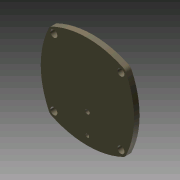
# Autodesk Inventor part: Between Seal 1764
Saved by Autodesk Inventor 2011 (Build 150239000, 239)
## iProperties
Created: 2010-01-18
Part Number: Between Seal 1764
Document SubType Name: Modeling
Designer: wbridges
Density: 1 g/cm^3
Author: wbridges
Autodesk Inventor part; units mm, degrees
ref_plane "YZ Plane" through (0, 0, 0) normal (1, 0, 0) x (0, 1, 0)
ref_plane "XZ Plane" through (0, 0, 0) normal (0, 1, 0) x (-1, 0, 0)
ref_plane "XY Plane" through (0, 0, 0) normal (0, 0, 1) x (1, 0, 0)
sketch "Sketch1" plane through (0, 0, 0) normal (0, 0, 1) x (1, 0, 0)
  circle A0 centre (-65.7225, 65.7225) radius 3.175
  circle A1 centre (-4.1275, 65.7225) radius 3.175
  circle A2 centre (-4.1275, 4.1275) radius 3.175
  circle A3 centre (-65.7225, 4.1275) radius 3.175
  arc A4 (-67.9183, -0.4854) -> (-1.9317, -0.4854) centre (-34.925, 68.8257) ccw
  arc A5 (-1.9317, 70.3354) -> (-67.9183, 70.3354) centre (-34.925, 1.0243) ccw
  arc A6 (-70.3354, 67.9183) -> (-70.3354, 1.9317) centre (-1.0243, 34.925) ccw
  arc A7 (0.4854, 1.9317) -> (0.4854, 67.9183) centre (-68.8257, 34.925) ccw
  circle A8 centre (-65.7225, 65.7225) radius 5.1089
  circle A9 centre (-4.1275, 65.7225) radius 5.1089
  circle A10 centre (-65.7225, 4.1275) radius 5.1089
  circle A11 centre (-4.1275, 4.1275) radius 5.1089
  arc A12 (-69.85, 62.7118) -> (-69.85, 7.1382) centre (-1.0243, 34.925) ccw
  arc A13 (-7.1382, 69.85) -> (-62.7118, 69.85) centre (-34.925, 1.0243) ccw
  arc A14 (0, 7.1382) -> (0, 62.7118) centre (-68.8257, 34.925) ccw
  arc A15 (-62.7118, 0) -> (-7.1382, 0) centre (-34.925, 68.8257) ccw
  point P0 (0, 0)
  point P1 (-34.925, 77.7875)
  point P2 (-34.925, -7.9375)
  point P3 (-77.7875, 34.925)
  point P4 (7.9375, 34.925)
  point P5 (-34.925, 77.7875)
  point P6 (-34.925, -7.9375)
  dimension "d36" = 6.35
  dimension "d37" = 61.595
  dimension "d38" = 61.595
  dimension "d39" = 85.725
  dimension "d40" = 2.54
  dimension "d41" = 2.54
  dimension "d42" = 2.54
  dimension "d43" = 2.54
  dimension "d44" = 67.8014
  dimension "d45" = 67.8014
  constraints: 36 point on circle, 16 centre point, 7 tangent, 6 coincident, 6 equal radius, 4 horizontal alignment, 4 vertical alignment
  measures "d36" diameter of A0
  measures "d37" distance of A1.centre A0.centre
  measures "d38" distance of A3.centre A0.centre
  measures "d39" distance of point (-34.925, -7.937) point (-34.925, 77.788)
  measures "d40" radial gap between concentric circles of A5 A13
  measures "d41" radial gap between concentric circles of A7 A14
  measures "d42" radial gap between concentric circles of A15 A4
  measures "d43" radial gap between concentric circles of A6 A12
  measures "d44" distance of A13.centre A15.centre
  measures "d45" distance of A12.centre A14.centre
extrude "Extrusion1" add sketch "Sketch1" along normal blind 5.08
sketch "Sketch2" plane through (0, 0, 0) normal (0, 0, -1) x (-1, 0, 0)
  circle A0 centre (34.925, 25.4) radius 17.78
  circle A1 centre (34.925, 25.4) radius 15.875
  circle A2 centre (34.925, 19.05) radius 2.0638
  circle A3 centre (34.925, 0) radius 1.5875
  circle A4 centre (34.925, 36.195) radius 4.445
  line L0 (34.925, 40.64) -> (34.925, 31.75)
  circle A5 centre (4.1275, 4.1275) radius 3.175 projected
  circle A6 centre (65.7225, 4.1275) radius 3.175 projected
  circle A7 centre (4.1275, 65.7225) radius 3.175 projected
  circle A8 centre (65.7225, 65.7225) radius 3.175 projected
  arc A9 (1.9317, -0.4854) -> (67.9183, -0.4854) centre (34.925, 68.8257) ccw projected
  arc A10 (67.9183, -0.4854) -> (70.3354, 1.9317) centre (65.7225, 4.1275) ccw projected
  arc A11 (70.3354, 1.9317) -> (70.3354, 67.9183) centre (1.0243, 34.925) ccw projected
  arc A12 (70.3354, 67.9183) -> (67.9183, 70.3354) centre (65.7225, 65.7225) ccw projected
  arc A13 (67.9183, 70.3354) -> (1.9317, 70.3354) centre (34.925, 1.0243) ccw projected
  arc A14 (1.9317, 70.3354) -> (-0.4854, 67.9183) centre (4.1275, 65.7225) ccw projected
  arc A15 (-0.4854, 67.9183) -> (-0.4854, 1.9317) centre (68.8257, 34.925) ccw projected
  arc A16 (-0.4854, 1.9317) -> (1.9317, -0.4854) centre (4.1275, 4.1275) ccw projected
  line L1 (50.8794, 25.4) -> (50.8794, 6.1059) projected
  arc A17 (50.8794, 25.4) -> (18.9706, 25.4) centre (34.925, 25.4) ccw projected
  line L2 (18.9706, 6.1059) -> (18.9706, 25.4) projected
  spline S0 degree 3 poles (14.9225, 8.7528) (15.0016, 8.6923) (15.081, 8.6322) (15.1606, 8.5725) (15.5075, 8.3124) (15.8596, 8.059) (16.5735, 7.5663) (16.9354, 7.3271) (17.3017, 7.0951) (17.668, 6.8631) (18.039, 6.6383) (18.5987, 6.3141) (18.7842, 6.2091) (18.9706, 6.1059) knots -0.55013 -0.55013 -0.55013 -0.55013 -0.52027 -0.52027 -0.52027 -0.390203 -0.390203 -0.260135 -0.260135 -0.260135 -0.130068 -0.130068 -0.066158 -0.066158 -0.066158 -0.066158 projected
  line L3 (14.9225, 8.7528) -> (14.9225, 25.4) projected
  arc A18 (54.9275, 25.4) -> (14.9225, 25.4) centre (34.925, 25.4) ccw projected
  line L4 (54.9275, 25.4) -> (54.9275, 8.7528) projected
  spline S1 degree 3 poles (50.8794, 6.1059) (51.0658, 6.2091) (51.2512, 6.3141) (51.811, 6.6383) (52.182, 6.8631) (52.5483, 7.0951) (52.9146, 7.3271) (53.2764, 7.5663) (53.9904, 8.059) (54.3425, 8.3124) (54.6894, 8.5725) (54.769, 8.6322) (54.8484, 8.6923) (54.9275, 8.7528) knots -0.454112 -0.454112 -0.454112 -0.454112 -0.390203 -0.390203 -0.260135 -0.260135 -0.260135 -0.130068 -0.130068 0 0 0 0.029861 0.029861 0.029861 0.029861 projected
  point P0 (34.925, 36.195)
  dimension "d10" = 1.905
  dimension "d11" = 35.56
  dimension "d15" = 4.1275
  dimension "d18" = 3.175
  dimension "d19" = 19.05
  dimension "d21" = 17.145
  dimension "d22" = 8.89
  dimension "d46" = 10.795
  dimension "d47" = 6.35
  constraints: 5 centre point, 3 vertical alignment, 2 coincident, 2 end point, 2 point on circle, 1 midpoint, 1 vertical
  measures "d10" radial gap between concentric circles of A1 A0
  measures "d11" diameter of A0
  measures "d15" diameter of A2
  measures "d18" diameter of A3
  measures "d19" distance of A2.centre A3.centre
  measures "d21" distance of A2.centre A4.centre
  measures "d22" diameter of A4
  measures "d46" distance of A0.centre A4.centre
  measures "d47" distance of A2.centre A0.centre
extrude "Extrusion2" cut sketch "Sketch2" against normal blind 2.54 contours A0 L1 A17 L2 | L2 A17 L1 A0
extrude "Extrusion3" cut sketch "Sketch2" along normal through all both and the other way through all contours A2 | A3
revolve "Revolution1" cut sketch "Sketch2" angle 360 about axis through (-34.925, 40.64, 0) along (0, -1, 0) picked at (34.5704, 34.7564) contours L0 A4
body "Solid1"
